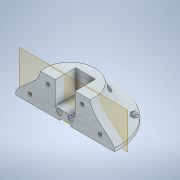
# Autodesk Inventor part: Podstawa 01-2
Saved by Autodesk Inventor 2021 (Build 250183000, 183)
## iProperties
Created: 2021-11-03
Part Number: Podstawa 01-2
Material: Generic
Document SubType Name: Modeling
Designer: Łukasz
Density: 1 g/cm^3
Appearance: Wood - Painted White
Author: Łukasz
Autodesk Inventor part; units mm, degrees
ref_plane "YZ Plane" through (0, 0, 0) normal (1, 0, 0) x (0, 1, 0)
ref_plane "XZ Plane" through (0, 0, 0) normal (0, 1, 0) x (-1, 0, 0)
ref_plane "XY Plane" through (0, 0, 0) normal (0, 0, 1) x (1, 0, 0)
sketch "Sketch1" plane through (0, 0, 0) normal (0, 0, 1) x (1, 0, 0)
  line L0 (0, 0) -> (-75, 0)
  line L1 (0, 0) -> (0, 50)
  line L2 (0, 50) -> (-38, 50)
  line L3 (-75, 0) -> (-75, 5)
  spline S0 degree 3 poles (-38, 50) (-46.7224, 6.6996) (-125.1064, 18.5226) (-28.5296, -55.0422) knots 0 0 0 0 1 1 1 1
  point P0 (-58.1914, 22.009)
  dimension "d0" = 75
  dimension "d1" = 50
  dimension "d2" = 38
  dimension "d3" = 5
  constraints: 8 end point, 2 horizontal, 2 vertical, 4 other
  measures "d0" distance of L0.start L0.end
  measures "d1" distance of L0.start L1.end
  measures "d2" distance of L1.end L2.end
  measures "d3" distance of L0.end L3.end
revolve "Revolution1" add sketch "Sketch1" angle 360 about axis through (0, 0, 0) along (0, 1, 0)
sketch "Sketch2" plane through (0, 50, 0) normal (0, 1, 0) x (1, 0, 0)
  line L0 (-15, 24) -> (15, 24)
  line L1 (15, 24) -> (15, -24)
  line L2 (15, -24) -> (-15, -24)
  line L3 (-15, -24) -> (-15, 24)
  point P0 (0, 0)
  dimension "d5" = 30
  dimension "d6" = 48
  dimension "d7" = 24
  dimension "d8" = 15
  constraints: 8 end point, 2 parallel, 1 horizontal, 1 perpendicular
  measures "d5" distance of L1.end L2.end
  measures "d6" distance of L0.end L1.end
  measures "d7" distance from line of point (0, 0) L0
  measures "d8" distance from line of L3 point (0, 0)
extrude "Extrusion1" cut sketch "Sketch2" against normal blind 35
sketch "Sketch3" plane through (0, 15, 0) normal (0, 1, 0) x (1, 0, 0)
  line L0 (15, -24) -> (-15, -24) projected
  line L1 (-15, -24) -> (-15, 24) projected
  line L2 (15, -24) -> (-15, -24)
  line L3 (-15, -24) -> (-15, -7)
  line L4 (-15, -7) -> (15, -7)
  line L5 (15, -7) -> (15, -24)
  point P0 (0, 0)
  dimension "d11" = 17
  constraints: 8 end point, 2 parallel, 1 horizontal, 1 perpendicular, 1 point on line
  measures "d11" distance of L2.end L3.end
extrude "Extrusion2" cut sketch "Sketch3" against normal blind 8
sketch "Sketch4" plane through (0, 0, 0) normal (0, 0, 1) x (1, 0, 0)
  circle A0 centre (-26, 38) radius 2.6
  circle A1 centre (-53, 12) radius 2.6
  line L0 (75, 0) -> (-75, 0) projected
  line L1 (38, 50) -> (-38, 50) projected
  line L2 (-75, 0) -> (-75, 5) projected
  line L3 (15, 50) -> (-15, 50) construction
  line L4 (0, 50) -> (0, 20.8019) construction
  circle A2 centre (26, 38) radius 2.6
  circle A3 centre (53, 12) radius 2.6
  point P0 (0, 0)
  dimension "d14" = 5.2
  dimension "d15" = 5.2
  dimension "d16" = 12
  dimension "d17" = 12
  dimension "d18" = 22
  dimension "d19" = 12
  constraints: 4 centre point, 2 end point, 2 symmetric about line, 1 midpoint, 1 vertical, 2 other
  measures "d14" diameter of A0
  measures "d15" diameter of A1
  measures "d16" distance from line of L0 A1.centre
  measures "d17" distance from line of L1 A0.centre
  measures "d18" distance from line of L2 A1.centre
  measures "d19" horizontal distance of L1.end A0.centre
extrude "Extrusion3" cut sketch "Sketch4" along normal blind 52 and the other way blind 52
ref_plane "Work Plane1" through (-15, 15, 7) normal (0, 0, 1) x (1, 0, 0)
split "Split1" plane through (-15, 15, 7) removes the side toward (0, 0, 1)
sketch "Sketch6" plane through (0, 0, 0) normal (0, -1, 0) x (1, 0, 0)
  circle A0 centre (0, 0) radius 10.5
  dimension "d25" = 21
  constraints: 1 centre point, 1 coincident
  measures "d25" diameter of A0
extrude "Extrusion4" cut sketch "Sketch6" against normal blind 2.5
ref_plane "Work Plane2" through (-15, 15, -5.5) normal (0, 0, 1) x (1, 0, 0)
sketch "Sketch7" plane through (-15, 15, -5.5) normal (0, 0, 1) x (1, 0, 0)
  circle A0 centre (41, 23) radius 2.6 projected
  line L0 (38.6906, 27) -> (43.3094, 27)
  line L1 (43.3094, 27) -> (45.6188, 23)
  line L2 (45.6188, 23) -> (43.3094, 19)
  line L3 (43.3094, 19) -> (38.6906, 19)
  line L4 (38.6906, 19) -> (36.3812, 23)
  line L5 (36.3812, 23) -> (38.6906, 27)
  circle A1 centre (-11, 23) radius 2.6 projected
  line L6 (-13.3094, 27) -> (-8.6906, 27)
  line L7 (-8.6906, 27) -> (-6.3812, 23)
  line L8 (-6.3812, 23) -> (-8.6906, 19)
  line L9 (-8.6906, 19) -> (-13.3094, 19)
  line L10 (-13.3094, 19) -> (-15.6188, 23)
  line L11 (-15.6188, 23) -> (-13.3094, 27)
  circle A2 centre (-38, -3) radius 2.6 projected
  line L12 (-35.6906, 1) -> (-33.3812, -3)
  line L13 (-33.3812, -3) -> (-35.6906, -7)
  line L14 (-35.6906, -7) -> (-40.3094, -7)
  line L15 (-40.3094, -7) -> (-42.6188, -3)
  line L16 (-42.6188, -3) -> (-40.3094, 1)
  line L17 (-40.3094, 1) -> (-35.6906, 1)
  circle A3 centre (68, -3) radius 2.6 projected
  line L18 (65.6906, 1) -> (70.3094, 1)
  line L19 (70.3094, 1) -> (72.6188, -3)
  line L20 (72.6188, -3) -> (70.3094, -7)
  line L21 (70.3094, -7) -> (65.6906, -7)
  line L22 (65.6906, -7) -> (63.3812, -3)
  line L23 (63.3812, -3) -> (65.6906, 1)
  line L24 (30, 35) -> (52.3497, 35) projected
  line L25 (-22.3497, 35) -> (0, 35) projected
  point P0 (15, -15)
  dimension "d29" = 8
  dimension "d30" = 8
  dimension "d31" = 8
  dimension "d32" = 8
  constraints: 48 end point, 4 coincident, 4 parallel, 52 other
  measures "d29" distance between parallel lines of L3 L0
  measures "d30" distance between parallel lines of L9 L6
  measures "d31" distance between parallel lines of L14 L17
  measures "d32" distance between parallel lines of L21 L18
extrude "Extrusion5" cut sketch "Sketch7" against normal blind 50 contours A0 | L0 L1 L2 L3 L4 L5 | A1 | L6 L7 L8 L9 L10 L11 | A2 | L12 L13 L14 L15 L16 L17 | A3 | L18 L19 L20 L21 L22 L23
sketch "Sketch8" plane through (-15, 15, 7) normal (0, 0, 1) x (1, 0, 0)
  point P0 (15, -15)
sketch "Sketch9" plane through (-15, 15, 7) normal (0, 0, 1) x (1, 0, 0)
  arc A0 (8.3697, -6.5166) -> (4.6303, -6.5166) centre (6.5, -4.5) ccw
  arc A1 (25.3697, -6.5166) -> (22.2084, -6.9278) centre (23.5, -4.5) ccw
  circle A2 centre (6.5, -4.5) radius 4.25
  circle A3 centre (23.5, -4.5) radius 4.25
  line L0 (7.1738, -15) -> (-59.6726, -15)
  spline S0 degree 3 poles (-59.6726, -10) (-58.7689, -7.9323) (-57.4468, -6.0708) (-54.3242, -2.5217) (-52.3894, -0.7667) (-46.4805, 4.2144) (-41.726, 7.6418) (-33.4997, 14.92) (-30.0416, 18.5511) (-24.9099, 26.5974) (-23.2478, 30.6178) (-22.3497, 35) knots -6.163162 -6.163162 -6.163162 -6.163162 -5.426539 -5.426539 -4.614235 -4.614235 -2.856788 -2.856788 -1.341997 -1.341997 0 0 0 0
  line L1 (-59.6726, -15) -> (-59.6726, -10)
  line L2 (-22.3497, 35) -> (0, 35)
  spline S1 degree 3 poles (52.3497, 35) (53.0647, 31.5111) (54.27, 28.2261) (57.5622, 22.1809) (59.5109, 19.5298) (66.0487, 12.2093) (71.1762, 8.2595) (79.7672, 1.4925) (83.3346, -1.3766) (87.4881, -6.1291) (88.7829, -7.9645) (89.6726, -10) knots -5.079654 -5.079654 -5.079654 -5.079654 -4.231884 -4.231884 -3.44283 -3.44283 -1.900227 -1.900227 -0.666449 -0.666449 0 0 0 0
  line L3 (30, 35) -> (52.3497, 35)
  line L4 (89.6726, -10) -> (89.6726, -15)
  line L5 (89.6726, -15) -> (22.8262, -15)
  point P0 (15, -15)
  dimension "d35" = 8.5
  dimension "d36" = 8.5
  constraints: 12 end point, 4 centre point, 4 point on circle, 2 coincident, 4 other
  measures "d35" diameter of A2
  measures "d36" diameter of A3
extrude "Extrusion6" cut sketch "Sketch9" against normal blind 1
sketch "Sketch10" plane through (-8.5, 10.5, 6) normal (0, 0, 1) x (1, 0, 0)
  circle A0 centre (0, 0) radius 0.75
  circle A1 centre (17, 0) radius 4.25 projected
  circle A2 centre (17, 0) radius 0.75
  point P0 (8.5, -10.5)
  dimension "d39" = 1.5
  dimension "d40" = 1.5
  constraints: 2 centre point, 1 coincident
  measures "d39" diameter of A0
  measures "d40" diameter of A2
extrude "Extrusion7" cut sketch "Sketch10" against normal blind 10 contours A0 | A2
equation "\"d7\" = 0.5 * d6"
equation "\"d8\" = 0.5 * d5"
body "Solid1"
